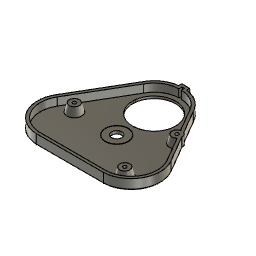
lense_turret_plastic_plate (Autodesk Fusion 360 design; units mm, degrees)
Autodesk Fusion 360 part; units mm, degrees
note: some values were not read from the file. Set by a fixed rule: which face or edge a step refers to.
sketch "Sketch1" plane through (0, 0, 0) normal (0, 0, 1) x (1, 0, 0)
  line L0 (0, 80) -> (0, -60) construction
  arc A0 (-3.5, 58.066445) -> (-22.511587, 44.977575) centre (-0.779866, 33.763847) ccw
  line L1 (-3.5, 58.066445) -> (-3.5, 61.099999)
  line L2 (-3.5, 61.099999) -> (0, 61.099999)
  line L3 (-22.511587, 44.977575) -> (-50.53947, -2.756371)
  line L4 (0, 61.099999) -> (3.5, 61.099999)
  line L5 (3.5, 61.099999) -> (3.5, 58.066445)
  arc A1 (22.511587, 44.977575) -> (3.5, 58.066445) centre (0.779866, 33.763847) ccw
  line L6 (22.511587, 44.977575) -> (50.53947, -2.756371)
  circle A2 centre (0, 32.894411) radius 19
  circle A3 centre (0, 0) radius 4.5
  circle A4 centre (-36.463554, -0.881949) radius 4.5
  circle A5 centre (34.737193, -27.636615) radius 4.5
  circle A6 centre (32.719466, 20.386653) radius 4.5
  circle A7 centre (32.719466, 20.386653) radius 3
  circle A8 centre (-36.463554, -0.881949) radius 3
  circle A9 centre (34.737193, -27.636615) radius 3
  circle A10 centre (32.719466, 20.386653) radius 1.5
  circle A11 centre (-36.463554, -0.881949) radius 1.5
  circle A12 centre (34.737193, -27.636615) radius 1.5
  circle A13 centre (0, 0) radius 10
  arc A14 (-50.53947, -2.756371) -> (-29.529259, -41.28179) centre (-28.472237, -15.713562) ccw
  arc A15 (29.529259, -41.28179) -> (50.53947, -2.756371) centre (28.472237, -15.713562) ccw
  line L7 (-29.529259, -41.28179) -> (0, -41.28179)
  line L8 (0, -41.28179) -> (29.529259, -41.28179)
  dimension "d3" = 38
  dimension "d4" = 9
  dimension "d32" = 9
  dimension "d34" = 9
  dimension "d36" = 9
  dimension "d42" = 6
  dimension "d43" = 6
  dimension "d44" = 6
  dimension "d47" = 3
  dimension "d48" = 3
  dimension "d49" = 3
  dimension "d52" = 20
  constraint vertical L0
  constraint parallel L0 L1
  constraint perpendicular L0 L2
  constraint perpendicular L0 L4
  constraint perpendicular L4 L5
  constraint coincident A3.centre A13.centre
  constraint concentric A6 A7
  constraint concentric A4 A8
  constraint concentric A5 A9
  constraint concentric A7 A10
  constraint concentric A4 A11
  constraint concentric A9 A12
  constraint concentric A3 A13
  constraint symmetric L0 A0 A1
  constraint symmetric L0 L3 L6
  constraint equal L3 L6
  constraint tangent L3 A14
  constraint symmetric L0 A14 A15
  constraint perpendicular L0 L7
  constraint symmetric L0 L7 L8
  measures "d3" diameter of A2
  measures "d4" diameter of A3
  measures "d32" diameter of A4
  measures "d34" diameter of A5
  measures "d36" diameter of A6
  measures "d42" diameter of A7
  measures "d43" diameter of A8
  measures "d44" diameter of A9
  measures "d47" diameter of A10
  measures "d48" diameter of A11
  measures "d49" diameter of A12
  measures "d52" diameter of A13
extrude "Extrude2" add sketch "Sketch1" along normal blind 9 contours A0 L1 L2 L3 L4 L5 A1 L6 A6 A14 A15 L7 L8 | L6 A6 | A4 | A5 | A7 | A8 | A9 | A10 | A11 | A12 | A13 picked at (11.296868, -26.075714) picked at (35.643288, 22.181608) picked at (-32.480307, -1.105513) picked at (38.720439, -27.860179) picked at (35.202712, 20.163089) picked at (-33.974723, -1.030992) picked at (37.220439, -27.860179) picked at (32.385507, 21.376694) picked at (-36.835664, -0.616384) picked at (35.103719, -27.296529) picked at (8.112682, -0.720371)
sketch "Sketch2" plane through (0, 0, 0) normal (0, 0, 1) x (1, 0, 0)
  line L0 (3.5, 61.099999) -> (3.5, 55.500001)
  line L1 (0, 61.099999) -> (3.5, 61.099999)
  line L2 (-3.5, 61.099999) -> (0, 61.099999)
  line L3 (-3.5, 55.500001) -> (-3.5, 61.099999)
  line L4 (3.5, 55.500001) -> (-3.5, 55.500001)
  constraint vertical L0
  constraint horizontal L2
sketch "Sketch3" plane through (0, 0, 9) normal (0, 0, 1) x (-1, 0, 0)
  arc A0 (-22.511587, -44.977575) -> (-3.5, -58.066445) centre (-0.779866, -33.763847) ccw
  line L0 (-3.5, -58.066445) -> (-3.5, -61.099999)
  line L1 (-3.5, -61.099999) -> (3.499997, -61.099999)
  line L2 (3.499997, -61.099999) -> (3.5, -58.066445)
  arc A1 (3.5, -58.066445) -> (22.511587, -44.977575) centre (0.779866, -33.763847) ccw
  line L3 (22.511587, -44.977575) -> (50.53947, 2.756371)
  circle A2 centre (0, -32.894411) radius 19
  circle A3 centre (0, 0) radius 4.5
  line L4 (22.511587, -44.977575) -> (50.53947, 2.756371)
  line L5 (-22.511587, -44.977575) -> (-50.53947, 2.756371)
  arc A4 (50.53947, 2.756371) -> (29.529259, 41.28179) centre (28.472237, 15.713562) ccw
  line L6 (29.529259, 41.28179) -> (-29.529259, 41.28179)
  arc A5 (-29.529259, 41.28179) -> (-50.53947, 2.756371) centre (-28.472237, 15.713562) ccw
  line L7 (-50.53947, 2.756371) -> (-22.511587, -44.977575)
  arc A6 (48.38363, 4.022213) -> (29.476277, 38.78179) centre (28.472237, 15.713562) ccw
  line L8 (29.476277, 38.78179) -> (-29.476277, 38.78179)
  arc A7 (-29.476277, 38.78179) -> (-48.38363, 4.022213) centre (-28.472237, 15.713562) ccw
  line L9 (-48.38363, 4.022213) -> (-20.320275, -43.772146)
  arc A8 (-20.320275, -43.772146) -> (-1, -55.717096) centre (-0.779866, -33.763847) ccw
  line L10 (-1, -55.717096) -> (-1, -58.599999)
  line L11 (-1, -58.599999) -> (1, -58.599999)
  line L12 (1, -58.599999) -> (1.000002, -55.717096)
  arc A9 (1.000002, -55.717096) -> (20.320275, -43.772146) centre (0.779866, -33.763847) ccw
  line L13 (20.320275, -43.772146) -> (48.38363, 4.022213)
  dimension "d81" = -2.5
extrude "Extrude7" add sketch "Sketch2" against normal blind 4 contours L0 L1 L2 L3 L4 picked at (0, 57.366667)
extrude "Extrude8" cut sketch "Sketch3" against normal blind 7 contours A3 | A6 L8 A7 L9 A8 L10 L11 L12 A9 L13 picked at (0.935235, 1.172747) picked at (0.112095, 27.350332)
extrude "Extrude11" add sketch "Sketch1" along normal blind 9 contours L6 A6 | L6 A6 | A4 | A5 | A7 | A8 | A9 | A10 | A11 | A12 picked at (36.308079, 21.975593) picked at (35.643288, 22.181608) picked at (-32.480307, -1.105513) picked at (38.720439, -27.860179) picked at (35.202712, 20.163089) picked at (-33.974723, -1.030992) picked at (37.220439, -27.860179) picked at (32.385507, 21.376694) picked at (-36.835664, -0.616384) picked at (35.103719, -27.296529)
extrude "Extrude12" cut sketch "Sketch1" along normal blind 6 contours A7 | A8 | A9 | A10 | A11 | A12 picked at (35.202712, 20.163089) picked at (-33.974723, -1.030992) picked at (37.220439, -27.860179) picked at (32.385507, 21.376694) picked at (-36.835664, -0.616384) picked at (35.103719, -27.296529)
extrude "Extrude13" cut sketch "Sketch1" along normal blind 9 contours A10 | A11 | A12 picked at (32.385507, 21.376694) picked at (-36.835664, -0.616384) picked at (35.103719, -27.296529)
extrude "Extrude14" add sketch "Sketch1" against normal blind 0.3 contours A13 picked at (8.112682, -0.720371)
sketch "Sketch4" plane through (0, 0, 2) normal (0, 0, 1) x (-1, 0, 0)
  arc A0 (-31.506968, -24.720225) -> (-35.913036, -17.216304) centre (-32.719466, -20.386653) ccw
  circle A1 centre (-34.737193, 27.636615) radius 4.5
  circle A2 centre (36.463554, 0.881949) radius 4.5
  circle A3 centre (0, 0) radius 4.5
  circle A4 centre (0, -32.894411) radius 19
  circle A5 centre (0, 0) radius 10
  line L0 (-31.506968, -24.720225) -> (-20.320275, -43.772146)
  arc A6 (-20.320275, -43.772146) -> (-1, -55.717096) centre (-0.779866, -33.763847) ccw
  line L1 (-1, -55.717096) -> (-1, -58.599999)
  line L2 (-1, -58.599999) -> (1.000001, -58.599999)
  line L3 (1, -58.599999) -> (1.000002, -55.717096)
  arc A7 (1.000002, -55.717096) -> (20.320275, -43.772146) centre (0.779866, -33.763847) ccw
  line L4 (20.320275, -43.772146) -> (48.38363, 4.022213)
  arc A8 (48.38363, 4.022213) -> (29.476277, 38.78179) centre (28.472237, 15.713562) ccw
  line L5 (29.476277, 38.78179) -> (-29.476277, 38.78179)
  arc A9 (-29.476277, 38.78179) -> (-48.38363, 4.022213) centre (-28.472237, 15.713562) ccw
  line L6 (-48.38363, 4.022213) -> (-35.913036, -17.216304)
  dimension "d56" = 20
  constraint concentric A3 A5
  measures "d56" diameter of A5
extrude "Extrude15" add sketch "Sketch4" along normal blind 0.3 contours A5 picked at (8.112682, -0.720371)
chamfer "Chamfer1" distance 2 distance2 7 3 edges at (28.838954, 18.108137, 2) (-40.659027, 0.74532, 2) (30.54172, -26.009346, 2) measured on face at (0.2491, -29.178539, 2) measured on face at (0.2491, -29.178539, 2) measured on face at (0.2491, -29.178539, 2)
fillet "Fillet2" radius 0.3 10 edges at (3.5, 55.500001, -2) (0, 55.500001, -4) (3.5, 58.3, -4) (-3.5, 58.3, -4) (-3.5, 55.500001, -2) (0, 61.099999, -4) (-3.5, 61.099999, 4.5) (-3.5, 61.099999, -2) (3.5, 61.099999, 2.5) (0, 61.099999, 9)
fillet "Fillet4" radius 0.4 3 edges at (-39.260536, -1.966796, 0) (29.922484, 19.301806, 0) (31.940211, -28.721462, 0)
sketch "Sketch8" plane through (-36.378799, 21.360495, 0) normal (-0.862336, 0.506337, 0) x (-0.506337, -0.862336, 0)
  line L0 (27.966906, 9) -> (-27.387333, 9)
  line L1 (-27.387333, 9) -> (-27.387333, 0)
  line L2 (-8.646448, 3) -> (7.353552, 3) construction
  line L3 (7.353552, 3) -> (7.353552, 7) construction
  line L4 (7.353552, 7) -> (-8.646448, 7) construction
  line L5 (-8.646448, 7) -> (-8.646448, 3) construction
  line L6 (-27.387333, 0) -> (27.966906, 0)
  line L7 (27.966906, 0) -> (27.966906, 9)
  dimension "d76" = 4
  text T0 "LW-23" font "Arial" height 4 bold align left top in box 16 x 4 at (-8.646448, 3) x (1, 0) y (0, 1) spacing 1
extrude "Extrude16" add sketch "Sketch8" along normal blind 0.5 text T0
fillet "Fillet5" radius 0.1 5 faces at (-32.568265, 28.837654, 4.547067) (-34.355526, 25.793792, 4.750796) (-38.276814, 19.115493, 3.237381) (-40.039103, 16.114161, 5.154536) (-37.28118, 20.811146, 4.322419)
fillet "Fillet6" radius 1 9 edges at (28.521904, 34.741478, 0) (14.647199, 53.906152, 0) (-14.647199, 53.906152, 0) (-36.525528, 21.110602, 0) (-50.93854, -27.965778, 0) (0, -41.28179, 0) (36.599977, 22.665168, 0) (50.93854, -27.965778, 0) (43.869467, 8.60323, 0)
